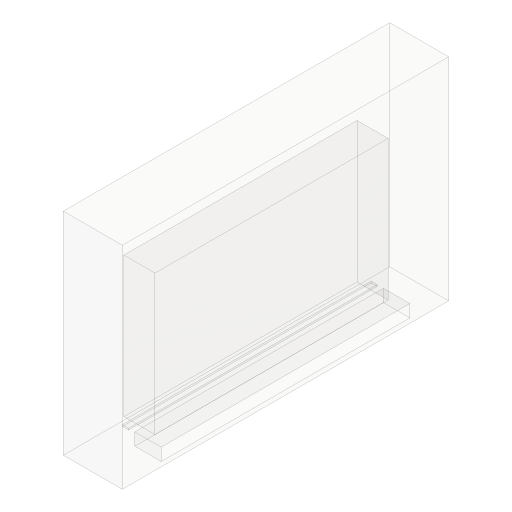
# Autodesk Inventor part: heater
Saved by Autodesk Inventor 2023 (Build 270158000, 158)
## iProperties
Created: 2022-09-09
Part Number: heater
Material: 聚碳酸酯，透明
Document SubType Name: Modeling
Designer: byfbi
Density: 1.2 g/cm^3
Appearance: 聚碳酸酯 - 透明
Author: byfbi
Autodesk Inventor part; units mm, degrees
sketch "草图1" plane through (0, 0, 0) normal (1, 0, 0) x (0, 1, 0)
  line L0 (340, -525) -> (-340, -525)
  line L1 (-340, -525) -> (-340, 525)
  line L2 (-340, 525) -> (340, 525)
  line L3 (340, 525) -> (340, -525)
  line L4 (340, -525) -> (-340, 525) construction
  line L5 (-340, -525) -> (340, 525) construction
  point P0 (0, 0)
  dimension "d0" = 680
  dimension "d1" = 1050
  constraints: 12 end point, 2 midpoint, 2 parallel, 1 horizontal, 1 perpendicular
  measures "d0" distance of L1.end L2.end
  measures "d1" distance of L0.end L1.end
extrude "拉伸1" add sketch "草图1" along normal blind 190
fillet "圆角1" [suppressed]
sketch "草图2" plane through (190, 0, 0) normal (1, 0, 0) x (0, 0, -1)
  line L0 (475, -290) -> (-475, -290) projected
  line L1 (475, 290) -> (475, -290) projected
  line L2 (-475, 290) -> (475, 290) projected
  line L3 (-475, -290) -> (-475, 290) projected
  line L4 (-475, 290) -> (475, 290)
  line L5 (475, 290) -> (475, 190)
  line L6 (475, 190) -> (-475, 190)
  line L7 (-475, 190) -> (-475, 290)
  point P0 (0, 0)
  dimension "d5" = 100
  constraints: 8 end point, 2 parallel, 1 horizontal, 1 perpendicular, 1 point on line
  measures "d5" distance of L4.end L5.end
extrude "拉伸2" [suppressed]
sketch "草图3" plane through (190, 0, 0) normal (1, 0, 0) x (0, 0, -1)
  line L0 (-475, -290) -> (-475, 290) projected
  line L1 (475, -290) -> (-475, -290) projected
  line L2 (475, 290) -> (475, -290) projected
  line L3 (-525, -340) -> (525, -340) projected
  line L4 (-525, 340) -> (-525, -340) projected
  line L5 (525, -340) -> (525, 340) projected
  line L6 (-475, -241.0052) -> (375, -241.0052)
  line L7 (375, -241.0052) -> (375, -341.0052)
  line L8 (375, -341.0052) -> (-475, -341.0052)
  line L9 (-475, -341.0052) -> (-475, -241.0052)
  point P0 (0, 0)
  point P1 (425, -191.0052)
  point P2 (425, -240)
  dimension "d8" = 850
  dimension "d9" = 100
  constraints: 8 end point, 2 parallel, 1 horizontal, 1 perpendicular, 1 point on line
  measures "d8" distance of L7.end L8.end
  measures "d9" distance of L6.end L7.end
extrude "拉伸3" [suppressed]
sketch "草图4" plane through (190, -191.0052, -425) normal (0, -1, 0) x (1, 0, 0)
  line L0 (-27.3454, 1.363) -> (-107.3454, 1.363)
  line L1 (-107.3454, 1.363) -> (-107.3454, 851.363)
  line L2 (-107.3454, 851.363) -> (-27.3454, 851.363)
  line L3 (-27.3454, 851.363) -> (-27.3454, 1.363)
  point P0 (-190, 425)
  dimension "d12" = 80
  dimension "d13" = 850
  constraints: 8 end point, 2 parallel, 1 horizontal, 1 perpendicular
  measures "d12" distance of L1.end L2.end
  measures "d13" distance of L0.end L1.end
extrude "拉伸4" [suppressed]
sketch "草图5" plane through (190, 0, 0) normal (1, 0, 0) x (0, 0, -1)
  line L0 (475, -290) -> (-475, -290) projected
  line L1 (475, 290) -> (475, -290) projected
  line L2 (-475, 290) -> (475, 290) projected
  line L3 (-475, -290) -> (-475, 290) projected
  line L4 (-400, -285) -> (400, -285)
  line L5 (400, -285) -> (400, -325)
  line L6 (400, -325) -> (-400, -325)
  line L7 (-400, -325) -> (-400, -285)
  line L8 (-525, -340) -> (525, -340) projected
  point P0 (0, 0)
  point P1 (-400, -305)
  point P2 (-400, -290)
  point P3 (400, -290)
  dimension "d16" = 800
  dimension "d17" = 40
  dimension "d19" = 75
  dimension "d34" = 55
  constraints: 8 end point, 2 parallel, 1 horizontal, 1 midpoint, 1 perpendicular
  measures "d16" distance of L5.end L6.end
  measures "d17" distance of L4.end L5.end
  measures "d19" distance from line of point (-400, -305) L3
  measures "d34" distance between parallel lines of L8 L4
extrude "拉伸5" cut sketch "草图5" against normal blind 105 contours L5 L6 L7 L0 | L0 L7 L4 L5
ref_plane "工作平面1" through (0, 165, 525) normal (0, 1, 0) x (1, 0, 0)
sketch "草图6" plane through (0, 165, 525) normal (0, 1, 0) x (1, 0, 0)
  line L0 (190, 50) -> (190, 1000) projected
  arc A0 (190, 1000) -> (140, 1050) centre (140, 1000) ccw projected
  line L1 (140, 1050) -> (140, 0) projected
  arc A1 (140, 0) -> (190, 50) centre (140, 50) ccw projected
  line L2 (0, 1050) -> (190, 1050) projected
  line L3 (0, 1050) -> (0, 0) projected
  line L4 (0, 0) -> (190, 0) projected
  line L5 (145, 150) -> (45, 150)
  line L6 (45, 150) -> (45, 900)
  line L7 (45, 900) -> (145, 900)
  line L8 (145, 900) -> (145, 150)
  line L9 (190, 1050) -> (190, 0) projected
  point P0 (0, 525)
  dimension "d23" = 100
  dimension "d24" = 750
  dimension "d25" = 150
  dimension "d26" = 45
  constraints: 8 end point, 2 parallel, 1 horizontal, 1 perpendicular
  measures "d23" distance of L6.end L7.end
  measures "d24" distance of L5.end L6.end
  measures "d25" distance between parallel lines of L2 L7
  measures "d26" distance between parallel lines of L3 L6
extrude "拉伸6" cut sketch "草图6" against normal blind 450 contours L5 L6 L7 L1 | L1 L7 L8 L5
fillet "圆角3" [suppressed]
ref_plane "工作平面2" through (0, -340, 225) normal (0, 0, 1) x (1, 0, 0)
sketch "草图7" plane through (0, -340, 225) normal (0, 0, 1) x (1, 0, 0)
  point P0 (0, 340)
sketch "草图8" plane through (0, -340, 225) normal (0, 0, 1) x (1, 0, 0)
  line L0 (-8.4267, 713.5838) -> (252.801, 713.5838)
  line L1 (252.801, 713.5838) -> (252.801, -46.692)
  line L2 (252.801, -46.692) -> (-8.4267, -46.692)
  line L3 (-8.4267, -46.692) -> (-8.4267, 713.5838)
  point P0 (0, 340)
  constraints: 8 end point, 2 parallel, 1 horizontal, 1 perpendicular
extrude "拉伸7" [suppressed]
sketch "草图9" plane through (190, -285, -400) normal (0, -1, 0) x (1, 0, 0)
  line L0 (0, 800) -> (-105, 800) projected
  line L1 (0, 0) -> (-105, 0) projected
  line L2 (-105, 0) -> (-105, 800) projected
  arc A0 (0, 875) -> (-50, 925) centre (-50, 875) ccw projected
  line L3 (0, 875) -> (-190, 875)
  line L4 (-190, -125) -> (-190, 925) projected
  arc A1 (-50, -125) -> (0, -75) centre (-50, -75) ccw projected
  line L5 (0, -75) -> (-190, -75)
  line L6 (-95, 875) -> (-95, -75)
  line L7 (-25, 800) -> (-65, 800)
  line L8 (-65, 800) -> (-65, 0)
  line L9 (-65, 0) -> (-25, 0)
  line L10 (-25, 0) -> (-25, 800)
  line L11 (-185, 800) -> (-145, 800)
  line L12 (-145, 800) -> (-145, 0)
  line L13 (-145, 0) -> (-185, 0)
  line L14 (-185, 0) -> (-185, 800)
  point P0 (-190, 400)
  point P1 (-14.2929, 800)
  point P2 (-14.2929, 0)
  point P3 (-25, 0)
  point P4 (-65, 800)
  dimension "d35" = 40
  dimension "d36" = 30
  constraints: 22 end point, 4 symmetric about line, 3 horizontal, 3 point on line, 2 midpoint, 2 parallel, 1 perpendicular
  measures "d35" distance between parallel lines of L8 L10
  measures "d36" distance between parallel lines of L6 L8
extrude "拉伸8" [suppressed]
ref_plane "工作平面3" through (125, 0, 0) normal (1, 0, 0) x (0, 0, -1)
sketch "草图10" plane through (125, 0, 0) normal (1, 0, 0) x (0, 0, -1)
  line L0 (400, -280) -> (-400, -280) projected
  line L1 (-400, -280) -> (-400, 220) projected
  line L2 (-400, 220) -> (400, 220) projected
  line L3 (400, -280) -> (400, 220) projected
  line L4 (-400, 220) -> (400, 220)
  line L5 (400, 220) -> (400, 160)
  line L6 (400, 160) -> (-400, 160)
  line L7 (-400, 160) -> (-400, 220)
  point P0 (0, 0)
  point P1 (-400, 160)
  point P2 (400, 160)
  dimension "d40" = 800
  dimension "d41" = 60
  constraints: 8 end point, 2 parallel, 1 horizontal, 1 perpendicular
  measures "d40" distance of L5.end L6.end
  measures "d41" distance of L4.end L5.end
extrude "拉伸9" [suppressed]
fillet "圆角4" [suppressed]
ref_plane "工作平面4" through (190, -290, -400) normal (0, -1, 0) x (1, 0, 0)
ref_plane "工作平面5" through (95, 0, 0) normal (1, 0, 0) x (0, 0, -1)
ref_plane "工作平面6" through (190, -290, 350) normal (0, 0, -1) x (-1, 0, 0)
sketch "草图11" plane through (0, -340, -525) normal (0, 0, -1) x (-1, 0, 0)
  point P0 (0, 340)
ref_plane "工作平面7" through (0, -340, 225) normal (0, 0, 1) x (1, 0, 0)
sketch "草图12" plane through (0, -340, 225) normal (0, 0, 1) x (1, 0, 0)
  line L0 (145, 505) -> (45, 505) projected
  line L1 (145, 55) -> (85, 55) projected
  line L2 (145, 505) -> (145, 55) projected
  line L3 (145, 505) -> (45, 505) projected
  line L4 (45, 505) -> (45, 55) projected
  line L5 (45, 55) -> (85, 55) projected
  line L6 (190, 55) -> (190, 15) projected
  line L7 (190, 55) -> (85, 55) projected
  line L8 (85, 55) -> (85, 15) projected
  line L9 (190, 15) -> (85, 15) projected
  line L10 (0, 0) -> (190, 0) projected
  line L11 (0, 0) -> (0, 680) projected
  line L12 (0, 680) -> (190, 680) projected
  line L13 (190, 0) -> (190, 680) projected
  point P0 (0, 340)
sketch "草图13" plane through (0, -340, -525) normal (0, 0, -1) x (-1, 0, 0)
  line L0 (-45, 505) -> (-45, 55) projected
  line L1 (-45, 55) -> (-85, 55) projected
  line L2 (-85, 55) -> (-85, 15) projected
  line L3 (-85, 55) -> (-65, 55)
  line L4 (-65, 55) -> (-65, 15)
  line L5 (-65, 15) -> (-85, 15)
  line L6 (-85, 15) -> (-85, 55)
  point P0 (0, 340)
  point P1 (-65, 35)
  dimension "d49" = 20
  dimension "d50" = 40
  dimension "d51" = 20
  constraints: 8 end point, 2 parallel, 1 horizontal, 1 midpoint, 1 perpendicular, 1 point on line
  measures "d49" distance of L4.end L5.end
  measures "d50" distance of L3.end L4.end
  measures "d51" distance from line of L0 point (-65, 35)
extrude "拉伸10" [suppressed]
sketch "草图14" plane through (190, -325, 400) normal (0, 0, -1) x (-1, 0, 0)
  line L0 (145, 490) -> (45, 490) projected
  line L1 (45, 490) -> (45, 40) projected
  line L2 (105, 40) -> (45, 40) projected
  line L3 (105, 40) -> (145, 40) projected
  line L4 (145, 490) -> (145, 40) projected
  line L5 (0, 40) -> (0, 0) projected
  line L6 (0, 40) -> (105, 40) projected
  line L7 (105, 40) -> (105, 0) projected
  line L8 (0, 0) -> (105, 0) projected
  line L9 (105, 40) -> (85, 40)
  line L10 (85, 40) -> (85, 0)
  line L11 (85, 0) -> (105, 0)
  line L12 (105, 0) -> (105, 40)
  line L13 (45, 40) -> (65, 40)
  line L14 (65, 40) -> (65, 20)
  line L15 (65, 20) -> (45, 20)
  line L16 (45, 20) -> (45, 40)
  line L17 (145, 40) -> (105, 40) projected
  line L18 (105, 40) -> (125, 40)
  line L19 (125, 40) -> (125, 35)
  line L20 (125, 35) -> (105, 35)
  line L21 (105, 35) -> (105, 40)
  point P0 (190, 325)
  point P1 (85, 40)
  dimension "d54" = 20
  dimension "d55" = 40
  dimension "d56" = 20
  dimension "d57" = 20
  dimension "d67" = 20
  dimension "d68" = 5
  constraints: 24 end point, 6 parallel, 3 horizontal, 3 perpendicular
  measures "d54" distance of L11.end L10.end
  measures "d55" distance of L10.end L9.end
  measures "d56" distance of L14.end L15.end
  measures "d57" distance of L13.end L14.end
  measures "d67" distance of L19.end L20.end
  measures "d68" distance of L18.end L19.end
extrude "拉伸11" add sketch "草图14" along normal blind 800 contours L2 L14 L15 L16 | L7 L8 L10 L2
sketch "草图15" plane through (190, -325, 400) normal (0, 0, -1) x (-1, 0, 0)
  line L0 (0, 40) -> (45, 40) projected
  line L1 (45, 40) -> (0, 40)
  line L2 (0, 40) -> (0, 35)
  line L3 (0, 35) -> (45, 35)
  line L4 (45, 35) -> (45, 40)
  point P0 (190, 325)
  dimension "d60" = 45
  dimension "d61" = 5
  constraints: 8 end point, 2 parallel, 1 horizontal, 1 perpendicular
  measures "d60" distance of L3.end L2.end
  measures "d61" distance of L2.end L1.end
extrude "拉伸12" [suppressed]
sketch "草图16" plane through (190, -325, 400) normal (0, 1, 0) x (1, 0, 0)
  line L0 (-105, 800) -> (-105, 0) projected
  line L1 (0, 800) -> (0, 0) projected
  line L2 (-105, 0) -> (0, 0)
  line L3 (0, 0) -> (0, 800)
  line L4 (0, 800) -> (-105, 800)
  line L5 (-105, 800) -> (-105, 0)
  point P0 (-190, 400)
  constraints: 8 end point, 2 parallel, 1 horizontal, 1 perpendicular
extrude "拉伸13" [suppressed]
fillet "圆角5" [suppressed]
sketch "草图17" plane through (190, -325, 400) normal (0, 0, -1) x (-1, 0, 0)
  line L0 (145, 40) -> (85, 40) projected
  line L1 (125, 40) -> (105, 40)
  line L2 (105, 40) -> (105, 35)
  line L3 (105, 35) -> (125, 35)
  line L4 (125, 35) -> (125, 40)
  line L5 (145, 490) -> (145, 40) projected
  point P0 (190, 325)
  point P1 (125, 37.5)
  point P2 (105, 40)
  dimension "d69" = 20
  dimension "d70" = 5
  dimension "d71" = 20
  constraints: 8 end point, 2 parallel, 1 horizontal, 1 midpoint, 1 perpendicular, 1 point on line
  measures "d69" distance of L3.end L2.end
  measures "d70" distance of L2.end L1.end
  measures "d71" distance from line of point (125, 37.5) L5
extrude "拉伸14" cut sketch "草图17" along normal blind 800
ref_plane "工作平面8" through (0, -340, 225) normal (0, 0, 1) x (1, 0, 0)
sketch "草图18" plane through (0, -340, 225) normal (0, 0, 1) x (1, 0, 0)
  line L0 (-8.4988, 711.8216) -> (199.7213, 711.8216)
  line L1 (199.7213, 711.8216) -> (199.7213, -36.0709)
  line L2 (199.7213, -36.0709) -> (-8.4988, -36.0709)
  line L3 (-8.4988, -36.0709) -> (-8.4988, 711.8216)
  point P0 (0, 340)
  constraints: 8 end point, 2 parallel, 1 horizontal, 1 perpendicular
extrude "拉伸15" [suppressed]
sketch "草图19" plane through (145, -305, 400) normal (1, 0, 0) x (0, 0, -1)
  line L0 (0, 20) -> (25, 20) projected
  line L1 (0, 0) -> (800, 0) projected
  line L2 (0, 20) -> (800, 20)
  line L3 (800, 20) -> (800, 0)
  line L4 (800, 0) -> (0, 0)
  line L5 (0, 0) -> (0, 20)
  point P0 (400, 305)
  constraints: 8 end point, 2 parallel, 1 horizontal, 1 perpendicular
extrude "拉伸16" [suppressed]
sketch "草图20" plane through (190, -325, 400) normal (0, 0, -1) x (-1, 0, 0)
  line L0 (65, 40) -> (85, 40) projected
  line L1 (65, 20) -> (45, 20) projected
  line L2 (65, 40) -> (45, 40)
  line L3 (45, 40) -> (45, 20)
  line L4 (45, 20) -> (65, 20)
  line L5 (65, 20) -> (65, 40)
  point P0 (190, 325)
  constraints: 8 end point, 2 parallel, 1 horizontal, 1 perpendicular
extrude "拉伸17" cut sketch "草图20" along normal blind 800
